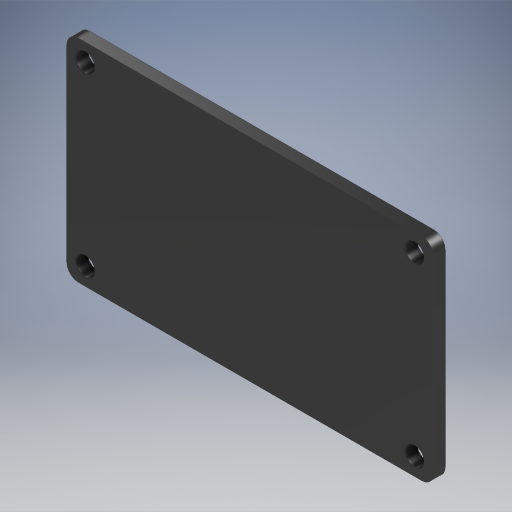
# Autodesk Inventor part: Limelight
Saved by Autodesk Inventor 2024.2 (Build 282272000, 272)
## iProperties
Created: 2024-02-01
Part Number: Limelight
Material: Generic
Document SubType Name: Modeling
Designer: rohan
Density: 1 g/cm^3
Appearance: Default
Author: rohan
Autodesk Inventor part; units mm, degrees
ref_plane "YZ Plane" through (0, 0, 0) normal (1, 0, 0) x (0, 1, 0)
ref_plane "XZ Plane" through (0, 0, 0) normal (0, 1, 0) x (-1, 0, 0)
ref_plane "XY Plane" through (0, 0, 0) normal (0, 0, 1) x (1, 0, 0)
sketch "Sketch1" plane through (0, 0, 0) normal (0, 0, 1) x (1, 0, 0)
  circle A0 centre (-44.4686, 23.8242) radius 2.5654
  circle A1 centre (44.4314, 23.8242) radius 2.5654
  line L0 (0, 25.1324) -> (0, 21.8881) construction
  circle A2 centre (-44.4686, -23.8008) radius 2.5654
  circle A3 centre (44.4314, -23.8008) radius 2.5654
  line L1 (44.4314, 23.8242) -> (44.4314, -23.8008)
  line L2 (-49.53, -28.575) -> (49.53, -28.575)
  line L3 (49.53, -28.575) -> (49.53, 28.575)
  line L4 (49.53, 28.575) -> (-49.53, 28.575)
  line L5 (-49.53, 28.575) -> (-49.53, -28.575)
  line L6 (-49.53, -28.575) -> (49.53, 28.575) construction
  line L7 (49.53, -28.575) -> (-49.53, 28.575) construction
  point P0 (0, 0)
  dimension "d0" = 5.1308
  dimension "d1" = 5.1308
  dimension "d2" = 88.9
  dimension "d5" = 47.625
  dimension "d10" = 99.06
  dimension "d11" = 57.15
  constraints: 16 end point, 4 centre point, 3 vertical, 2 midpoint, 2 parallel, 1 horizontal, 1 perpendicular, 4 other
  measures "d0" diameter of A0
  measures "d1" diameter of A1
  measures "d2" distance of A0.centre L1.start
  measures "d5" distance of A0.centre A2.centre
  measures "d10" distance of L4.end L3.end
  measures "d11" distance of L3.end L2.end
extrude "Extrusion1" add sketch "Sketch1" along normal blind 3.175
fillet "Fillet1" radius 3.175 4 edges at (-49.53, 28.575, 1.5875) (49.53, 28.575, 1.5875) (49.53, -28.575, 1.5875) (-49.53, -28.575, 1.5875)
body "Solid1"
